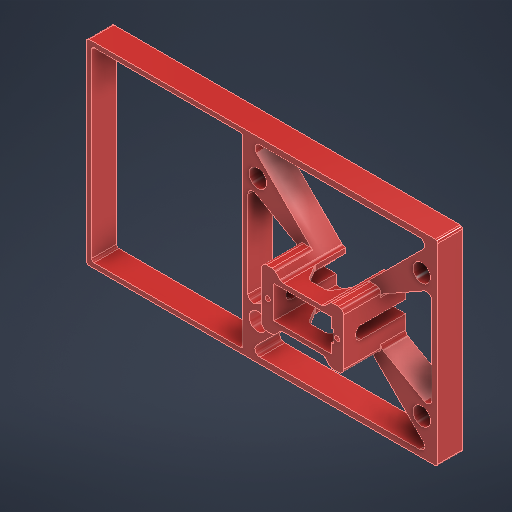
# Autodesk Inventor part: Servo_holder
Saved by Autodesk Inventor 2026.1 (Build 301233020, 233B)
## iProperties
Created: 2025-12-03
Part Number: Servo_holder
Material: Generic
Document SubType Name: Modeling
Designer: samuel
Density: 1 g/cm^3
Appearance: Orange-Red
Author: samuel
Autodesk Inventor part; units mm, degrees
ref_plane "YZ Plane" through (0, 0, 0) normal (1, 0, 0) x (0, 1, 0)
ref_plane "XZ Plane" through (0, 0, 0) normal (0, 1, 0) x (-1, 0, 0)
ref_plane "XY Plane" through (0, 0, 0) normal (0, 0, 1) x (1, 0, 0)
sketch "Sketch1" plane through (0, 0, 0) normal (0, 0, 1) x (1, 0, 0)
  line L0 (-37, -37) -> (37, -37)
  line L1 (37, -37) -> (37, 37)
  line L2 (37, 37) -> (-37, 37)
  line L3 (-37, 37) -> (-37, -37)
  line L4 (-37, -37) -> (37, 37) construction
  line L5 (37, -37) -> (-37, 37) construction
  line L6 (-39, 37.5) -> (-100, 37.5)
  line L7 (-100, 37.5) -> (-100, -37.5)
  line L8 (-100, -37.5) -> (-39, -37.5)
  line L9 (-39, -37.5) -> (-39, 37.5)
  line L10 (-102, 39.5) -> (-37, 39.5)
  line L11 (-37, 39.5) -> (-37, -39.5)
  line L12 (-37, -39.5) -> (-102, -39.5)
  line L13 (-102, -39.5) -> (-102, 39.5)
  line L14 (-39.5, 39.5) -> (39.5, 39.5)
  line L15 (39.5, 39.5) -> (39.5, -39.5)
  line L16 (39.5, -39.5) -> (-39.5, -39.5)
  line L17 (-11.5, 6.5) -> (11.5, 6.5)
  line L18 (11.5, 6.5) -> (11.5, -6.5)
  line L19 (11.5, -6.5) -> (-11.5, -6.5)
  line L20 (-11.5, -6.5) -> (-11.5, 6.5)
  line L21 (-11.5, 6.5) -> (11.5, -6.5) construction
  line L22 (11.5, 6.5) -> (-11.5, -6.5) construction
  line L23 (-37, -37) -> (-6.5, -6.5)
  line L24 (6.5, -6.5) -> (37, -37)
  line L25 (6.5, 6.5) -> (37, 37)
  line L26 (-6.5, 6.5) -> (-37, 37)
  line L27 (-11.5, 6.5) -> (-37, 20.913)
  line L28 (-11.5, -6.5) -> (-37, -20.913)
  line L29 (11.5, 6.5) -> (37, 20.913)
  line L30 (11.5, -6.5) -> (37, -20.913)
  line L31 (-13.5, -8.5) -> (13.5, -8.5)
  line L32 (13.5, -8.5) -> (13.5, 8.5)
  line L33 (13.5, 8.5) -> (-13.5, 8.5)
  line L34 (-13.5, 8.5) -> (-13.5, -8.5)
  line L35 (-13.5, -8.5) -> (13.5, 8.5) construction
  line L36 (13.5, -8.5) -> (-13.5, 8.5) construction
  line L37 (-16.5, -11.5) -> (16.5, -11.5)
  line L38 (16.5, -11.5) -> (16.5, 11.5)
  line L39 (16.5, 11.5) -> (-16.5, 11.5)
  line L40 (-16.5, 11.5) -> (-16.5, -11.5)
  point P0 (0, 0)
  point P1 (-39, 0)
  point P2 (-37, -20.913)
  point P3 (13.5, -7.6304)
  point P4 (13.5, 7.6304)
  point P5 (-13.5, -7.6304)
  point P6 (-13.5, 7.6304)
  point P7 (8.5, -8.5)
  point P8 (11.5, -11.5)
  point P9 (11.5, 11.5)
  point P10 (8.5, 8.5)
  point P11 (-11.5, -11.5)
  point P12 (-8.5, -8.5)
  point P13 (-8.5, 8.5)
  point P14 (-11.5, 11.5)
  dimension "d3" = 61
  dimension "d4" = 75
  dimension "d5" = 37.5
  dimension "d6" = 2
  dimension "d9" = 23
  dimension "d10" = 13
  dimension "d17" = 3
  constraints: 82 end point, 16 point on line, 13 parallel, 7 perpendicular, 6 midpoint, 4 horizontal, 3 collinear, 8 other
  measures "d3" distance of L8.end L7.end
  measures "d4" distance of L7.end L6.end
  measures "d5" distance from line of point (-39, 0) L8
  measures "d6" distance between parallel lines of L6 L10
  measures "d9" distance of L18.end L19.end
  measures "d10" distance of L17.end L18.end
  measures "d17" distance between parallel lines of L34 L40
extrude "Extrusion1" add sketch "Sketch1" along normal blind 10 contours L11 L12 L13 L10 L3 | L0 L1 L2 L11 L14 L15 L16 | L3 L28 L40 L37 L23 | L24 L37 L38 L30 L1 | L37 L40 L28 L34 L31 L23 | L24 L31 L32 L30 L38 L37 | L3 L26 L39 L40 L27 | L31 L34 L28 L19 L23 | L29 L38 L39 L25 L1 | L24 L19 L30 L32 L31 | L40 L39 L26 L33 L34 L27 | L29 L32 L33 L25 L39 L38 | L34 L33 L26 L17 L27 | L29 L17 L25 L33 L32
extrude "Extrusion2" add sketch "Sketch1" along normal blind 25 contours L37 L40 L28 L34 L31 L23 | L24 L31 L32 L30 L38 L37 | L40 L27 L34 L28 | L31 L34 L28 L19 L23 | L23 L19 L24 L31 | L30 L32 L29 L38 | L24 L19 L30 L32 L31 | L40 L39 L26 L33 L34 L27 | L34 L27 L20 L28 | L29 L32 L33 L25 L39 L38 | L30 L18 L29 L32 | L34 L33 L26 L17 L27 | L29 L17 L25 L33 L32 | L33 L25 L17 L26
sketch "Sketch3" plane through (0, 0, 25) normal (0, 0, 1) x (1, 0, 0)
  line L0 (11.5, 6.5) -> (11.5, -6.5) projected
  line L1 (11.5, 0) -> (12.5, 0)
  line L2 (12.5, 0) -> (12.5, 2.5)
  line L3 (12.5, 2.5) -> (11.5, 2.5)
  line L4 (11.5, 2.5) -> (11.5, 0)
  line L5 (12.5, 0) -> (12.5, -2.5)
  line L6 (12.5, -2.5) -> (11.5, -2.5)
  point P0 (0, 0)
  dimension "d18" = 1
  dimension "d19" = 2.5
  constraints: 12 end point, 2 parallel, 2 symmetric about line, 1 horizontal, 1 midpoint, 1 perpendicular
  measures "d18" distance of L3.end L2.end
  measures "d19" distance of L2.end L1.end
extrude "Extrusion3" cut sketch "Sketch3" against normal through all
sketch "Sketch4" plane through (0, 0, 0) normal (0, 0, -1) x (-1, 0, 0)
  line L0 (-12.5, -2.5) -> (-11.5, -2.5) projected
  line L1 (-16.5, -11.5) -> (-16.5, 11.5) projected
  line L2 (-12.5, -2.5) -> (-16.5, -2.5)
  line L3 (-16.5, -2.5) -> (-16.5, 2.5)
  line L4 (-16.5, 2.5) -> (-12.5, 2.5)
  line L5 (-12.5, 2.5) -> (-12.5, -2.5)
  point P0 (0, 0)
  dimension "d22" = 5
  constraints: 8 end point, 2 parallel, 1 horizontal, 1 perpendicular, 1 point on line
  measures "d22" distance of L2.end L3.end
extrude "Extrusion4" cut sketch "Sketch4" against normal blind 20
fillet "Fillet1" radius 2 24 edges at (-37, 20.913, 5) (-8.5, -8.5, 12.5) (8.5, -8.5, 12.5) (37, 20.913, 5) (37, 37, 5) (-37, 37, 5) (-37, -20.913, 5) (-37, -37, 5) (37, -37, 5) (37, -20.913, 5) (-8.5, 8.5, 12.5) (8.5, 8.5, 12.5) (11.5, -11.5, 17.5) (16.5, -11.5, 17.5) (-16.5, -11.5, 17.5) (-11.5, -11.5, 17.5) (-16.5, 11.5, 17.5) (-11.5, 11.5, 17.5) (11.5, 11.5, 17.5) (16.5, 11.5, 17.5) (16.5, 9.3261, 5) (16.5, -9.3261, 5) (-16.5, -9.3261, 5) (-16.5, 9.3261, 5)
fillet "Fillet2" radius 1 8 edges at (-39, 37.5, 5) (-39, -37.5, 5) (-100, -37.5, 5) (-100, 37.5, 5) (-102, 39.5, 5) (-102, -39.5, 5) (39.5, -39.5, 5) (39.5, 39.5, 5)
sketch "Sketch5" plane through (0, 0, 25) normal (0, 0, 1) x (1, 0, 0)
  circle A0 centre (-14, 0) radius 1
  line L0 (-11.5, -6.5) -> (-11.5, 6.5) projected
  circle A1 centre (14, 0) radius 1
  line L1 (16.5, -9.5) -> (16.5, 9.5) projected
  circle A2 centre (-33, 25) radius 3.5
  circle A3 centre (-33, -25) radius 3.5
  point P0 (0, 0)
  dimension "d31" = 2
  dimension "d32" = 2.5
  dimension "d33" = 2
  dimension "d34" = 2.5
  dimension "d37" = 7
  dimension "d38" = 7
  dimension "d39" = 50
  dimension "d40" = 33
  dimension "d41" = 25
  dimension "d42" = 0
  constraints: 4 centre point
  measures "d31" diameter of A0
  measures "d32" distance from line of L0 A0.centre
  measures "d33" diameter of A1
  measures "d34" distance from line of L1 A1.centre
  measures "d37" diameter of A2
  measures "d38" diameter of A3
  measures "d39" distance of A3.centre A2.centre
  measures "d40" horizontal distance of point (0, 0) A3.centre
  measures "d41" vertical distance of point (0, 0) A2.centre
  measures "d42" horizontal distance of A3.centre A2.centre
extrude "Extrusion5" cut sketch "Sketch5" against normal through all
mirror "Mirror1" about plane through (0, 0, 0) normal (1, 0, 0) of "Extrusion5"
sketch "Sketch6" plane through (-7.6716, -8.5, 0) normal (0, -1, 0) x (1, 0, 0)
  line L0 (0, 25) -> (0, 0) projected
  line L1 (15.3431, 0) -> (15.3431, 25) projected
  line L2 (0, 25) -> (15.3431, 25)
  line L3 (15.3431, 25) -> (15.3431, 0)
  line L4 (15.3431, 0) -> (0, 0)
  line L5 (0, 0) -> (0, 25)
  line L6 (0, 25) -> (15.3431, 0)
  line L7 (0, 0) -> (15.3431, 25)
  line L8 (7.6716, 12.5) -> (7.6716, 25)
  line L9 (7.6716, 12.5) -> (7.6716, 0)
  line L10 (7.6716, 12.5) -> (15.3431, 12.5)
  line L11 (15.3431, 25) -> (15.3431, 0) projected
  line L12 (7.6716, 12.5) -> (0, 12.5)
  line L13 (0, 12.5) -> (7.6716, 0)
  line L14 (15.3431, 12.5) -> (7.6716, 0)
  line L15 (15.3431, 12.5) -> (7.6716, 25)
  line L16 (0, 12.5) -> (7.6716, 25)
  line L17 (3.8358, 18.75) -> (11.5074, 18.75)
  constraints: 30 end point, 6 midpoint, 5 equal length, 1 horizontal, 1 perpendicular
extrude "Extrusion6" cut sketch "Sketch6" along normal mid plane 50 contours L13 L7 L0 | L16 L6 L12 | L12 L7 L13 | L17 L8 L6 | L7 L13 L4 | L10 L14 L6 | L8 L17 L7 | L9 L13 L7 | L6 L14 L9 | L7 L15 L10 | L14 L6 L4 | L14 L1 L6
sketch "Sketch8" plane through (-16.5, -8.1592, 0) normal (-1, 0, 0) x (0, 0, 1)
  line L0 (25, 10.6592) -> (20, 10.6592) projected
  line L1 (25, 10.6592) -> (-1.765, 10.6592)
  line L2 (-1.765, 10.6592) -> (-1.765, 5.6592)
  line L3 (-1.765, 5.6592) -> (25, 5.6592)
  line L4 (25, 5.6592) -> (25, 10.6592)
  line L5 (0, 16.3183) -> (0, 0) projected
  line L6 (0, 10.6592) -> (20, 10.6592)
  line L7 (20, 10.6592) -> (20, 5.6592)
  line L8 (20, 5.6592) -> (0, 5.6592)
  line L9 (0, 5.6592) -> (0, 10.6592)
  point P0 (0, 8.1592)
  point P1 (17.0858, 10.6592)
  dimension "d48" = 5
  dimension "d49" = 20
  constraints: 16 end point, 4 parallel, 3 point on line, 2 horizontal, 2 perpendicular
  measures "d48" distance of L2.end L1.end
  measures "d49" distance of L7.end L8.end
extrude "Extrusion7" cut sketch "Sketch8" against normal blind 10 contours L7 L3 L5 L1
fillet "Fillet6" radius 2 12 edges at (-14, -2.5, 20) (-14, 2.5, 20) (14.5, 2.5, 20) (14.5, -2.5, 20) (-3.8358, 7.5, 18.75) (3.8358, 7.5, 18.75) (-3.8358, -7.5, 18.75) (3.8358, -7.5, 18.75) (-7.6716, -7.5, 12.5) (-7.6716, 7.5, 12.5) (7.6716, 7.5, 12.5) (7.6716, -7.5, 12.5)
body "Solid1"
